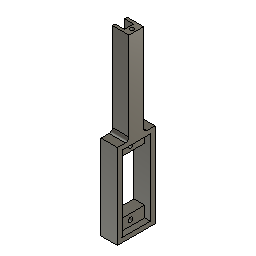
Polish cow v24 (Autodesk Fusion 360 archive; units mm, degrees)
design "Polish cow stand"
Autodesk Fusion 360 part; units mm, degrees
sketch "Sketch1" plane through (0, 0, 0) normal (1, 0, 0) x (0, 1, 0)
  line L0 (0, 0) -> (12.4, 0)
  line L1 (12.4, 0) -> (12.4, 23.4)
  line L2 (12.4, 23.4) -> (0, 23.4)
  line L3 (0, 23.4) -> (0, 0)
  line L4 (6.2, 23.4) -> (6.2, 32.8204) construction
  line L5 (0, 23.4) -> (12.4, 23.4)
  line L6 (12.4, 23.4) -> (12.4, 28.2)
  line L7 (12.4, 28.2) -> (0, 28.2)
  line L8 (0, 28.2) -> (0, 23.4)
  line L9 (0, 0) -> (12.4, 0)
  line L10 (12.4, 0) -> (12.4, -4.8)
  line L11 (12.4, -4.8) -> (0, -4.8)
  line L12 (0, -4.8) -> (0, 0)
  line L13 (-2, 30.2) -> (14.4, 30.2)
  line L14 (14.4, 30.2) -> (14.4, -6.8)
  line L15 (14.4, -6.8) -> (-2, -6.8)
  line L16 (-2, -6.8) -> (-2, 30.2)
  circle A0 centre (6.2, 25.65) radius 1
  line L17 (6.2, -4.8) -> (6.2, 0) construction
  circle A1 centre (6.2, -2.4) radius 1
  line L18 (3, 30.2) -> (3, 70.2)
  line L19 (-7.8, 50.2) -> (6, 50.2) construction
  line L20 (3, 50.2) -> (0, 50.2)
  line L21 (-7.8, 45.2) -> (6, 45.2) construction
  line L22 (4.2, 30.2) -> (4.2, 70.2)
  line L23 (3, 70.2) -> (4.2, 70.2)
  line L24 (4.2, 70.2) -> (6.2, 70.2)
  line L25 (8.2, 30.2) -> (8.2, 70.2)
  line L26 (9.4, 30.2) -> (9.4, 70.2)
  line L27 (8.2, 70.2) -> (6.2, 70.2)
  line L28 (9.4, 70.2) -> (8.2, 70.2)
  point P0 (20.2, 45.2)
  point P1 (20.2, 50.2)
  dimension "d2" = 23.4
  dimension "d6" = 4.8
  dimension "d7" = 12.4
  dimension "d8" = 12.4
  dimension "d10" = 4.8
  dimension "d16" = 2
  dimension "d17" = 2
  dimension "d18" = 2
  dimension "d19" = 2
  dimension "d20" = 2.25
  dimension "d21" = 2
  dimension "d22" = 2.4
  dimension "d23" = 2
  dimension "d24" = 40
  dimension "d25" = 3.2
  dimension "d26" = 20
  dimension "d27" = 3
  dimension "d28" = 5
  dimension "d30" = 1.2
  dimension "d31" = 2
  constraint horizontal L0
  constraint vertical L1
  constraint horizontal L2
  constraint vertical L3
  constraint coincident L0.start L3.end
  constraint midpoint L2 L4.start
  constraint perpendicular L2 L4
  constraint perpendicular L5 L6
  constraint parallel L5 L7
  constraint parallel L6 L8
  constraint horizontal L9
  constraint vertical L10
  constraint horizontal L11
  constraint vertical L12
  constraint horizontal L13
  constraint vertical L14
  constraint horizontal L15
  constraint vertical L16
  constraint coincident L4 A0.centre
  constraint midpoint L11 L17.start
  constraint midpoint L9 L17.end
  constraint midpoint L17 A1.centre
  constraint coincident L13 L18.start
  constraint perpendicular L13 L18
  constraint perpendicular L18 L19
  constraint coincident L18 L20.start
  constraint coincident L19 L20.start
  constraint perpendicular L18 L20
  constraint horizontal L21
  constraint coincident L13 L22.start
  constraint perpendicular L13 L22
  constraint perpendicular L22 L23
  constraint perpendicular L22 L24
  constraint symmetric L4 L18.start L26.start
  constraint symmetric L4 L18.end L26.end
  constraint symmetric L4 L19.start P1
  constraint symmetric L4 L21.start P0
  constraint symmetric L4 L22.start L25.start
  constraint symmetric L4 L22.end L25.end
  constraint symmetric L4 L24.end L27.end
  measures "d2" distance of L0.start L2.end
  measures "d6" distance of L0.end L10.end
  measures "d7" distance of L10.end L11.end
  measures "d8" distance of L1 L3
  measures "d10" distance of L5 L7
  measures "d16" distance of L3 L16
  measures "d17" distance of L1 L14
  measures "d18" distance of L7 L13
  measures "d19" distance of L11 L15
  measures "d20" distance of L2 A0.centre
  measures "d21" diameter of A1
  measures "d22" distance of L17.end A1.centre
  measures "d23" diameter of A0
  measures "d24" distance of L18.start L18.end
  measures "d25" distance of L4 L18
  measures "d26" distance of L18.end L19
  measures "d27" distance of L20.start L20.end
  measures "d28" distance of L20.start L21
  measures "d30" distance of L18 L22
  measures "d31" distance of L22.end L24.end
extrude "Extrude1" add sketch "Sketch1" along normal blind 3.2 contours L13 L18 L22 L23 | L13 L22 L24 L25 L27 | L13 L25 L26 L28 makes body 1
extrude "Extrude2" add sketch "Sketch1" against normal blind 4 contours L13 L18 L22 L23 | L13 L25 L26 L28 bodies 1
extrude "Extrude3" add sketch "Sketch1" along normal blind 3.2 contours L13 L14 L15 L16 bodies 1
extrude "Extrude4" add sketch "Sketch1" along normal blind 0.7 contours L0 L9 L10 L11 L12 | L2 L5 L6 L7 L8 bodies 1
extrude "Extrude5" add sketch "Sketch1" against normal blind 4 contours L0 L9 L10 L11 L12 | L2 L5 L6 L7 L8 | L13 L14 L15 L16 bodies 1
ref_plane "WorkPlane1" through (-4, 3.6, 50.2) normal (-1, 0, 0) x (0, 0, 1)
sketch "Sketch2" plane through (-4, 0, 0) normal (-1, 0, 0) x (0, -1, 0)
  line L0 (-8.2, 41.4) -> (-4.2, 41.4)
  line L1 (-4.2, 41.4) -> (-4.2, 40.2)
  line L2 (-4.2, 40.2) -> (-8.2, 40.2)
  line L3 (-8.2, 40.2) -> (-8.2, 41.4)
  line L4 (2, 30.2) -> (-14.4, 30.2)
  line L5 (-4.2, 58.4) -> (-4.2, 57.2)
  line L6 (-4.2, 57.2) -> (-8.2, 57.2)
  line L7 (-8.2, 57.2) -> (-8.2, 58.4)
  line L8 (-8.2, 58.4) -> (-4.2, 58.4)
  line L9 (-8.2, 30.2) -> (-4.2, 30.2)
  line L10 (-4.2, 30.2) -> (-4.2, 70.2)
  line L11 (-4.2, 70.2) -> (-8.2, 70.2)
  line L12 (-8.2, 70.2) -> (-8.2, 30.2)
  dimension "d43" = 1.2
  dimension "d44" = 10
  dimension "d47" = 0
  dimension "d48" = 34
  constraint horizontal L0
  constraint vertical L1
  constraint horizontal L2
  constraint vertical L3
  constraint coincident L2.end L12
  constraint coincident L0.end L10
  measures "d43" distance of L0.start L2.end
  measures "d44" distance of L2 L4
extrude "Extrude6" add sketch "Sketch2" against normal blind 0.8 contours L0 L1 L2 L3 L10 L12 | L5 L6 L7 L8 L10 L12 bodies 1
ref_plane "WorkPlane2" through (0, 0, 70.2) normal (0, 0, 1) x (1, 0, 0)
sketch "Sketch3" plane through (0, 0, 70.2) normal (0, 0, 1) x (1, 0, 0)
  line L0 (0, 6) -> (3.2, 6) construction
  circle A0 centre (1.6, 6) radius 0.9
  dimension "d52" = 3.2
  dimension "d53" = 1.8
  constraint horizontal L0
  constraint midpoint L0 A0.centre
  measures "d52" distance of L0.start L0.end
  measures "d53" diameter of A0
extrude "Extrude7" cut sketch "Sketch3" against normal blind 7 bodies 1
sketch "Sketch4" plane through (0, 0, 0) normal (1, 0, 0) x (0, 1, 0)
fillet "Fillet3" radius 1.5 2 edges at (-0.4, 3, 30.2) (-0.4, 9.4, 30.2) on bodies 1
copy_body "Body->Comp1" bodies 1 removing the originals makes body 2 in component "Stand"
component "Stand" placed x (1, 0, 0) y (0, 1, 0) z (0, 0, 1) at (0, 0, 0)
named bodies: "Stand"
